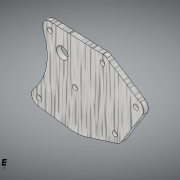
# Autodesk Inventor part: 後ろ脚内フレーム
Saved by Autodesk Inventor 2019 (Build 230136000, 136)
## iProperties
Created: 2019-09-18
Part Number: 後ろ脚内フレーム
Material: アルミニウム 7075
Document SubType Name: Modeling
Designer: tanjihayato
Density: 2.81 g/cm^3
Appearance: サテン - ブラシ仕上げ 重厚
Mass: 19.8491 g
Surface Area: 54.8854 cm^2
Volume: 7.06374 cm^3
Author: tanjihayato
Autodesk Inventor part; units mm, degrees
ref_plane "YZ Plane" through (0, 0, 0) normal (1, 0, 0) x (0, 1, 0)
ref_plane "XZ Plane" through (0, 0, 0) normal (0, 1, 0) x (-1, 0, 0)
ref_plane "XY Plane" through (0, 0, 0) normal (0, 0, 1) x (1, 0, 0)
sketch "スケッチ1" plane through (0, 0, 0) normal (0, 0, 1) x (1, 0, 0)
  circle A0 centre (-21.6908, -16.4118) radius 19.1 construction
  circle A1 centre (-58.0056, -24.4791) radius 22.1 construction
  circle A2 centre (-105.5257, -16.4118) radius 30.1 construction
  circle A3 centre (-122.6945, 30.2622) radius 1.5
  circle A4 centre (-75.5257, 23.124) radius 1.5
  circle A5 centre (-65.5257, -10.4118) radius 1.5
  circle A6 centre (-145.5257, 0.5882) radius 1.5
  circle A7 centre (-105.5257, -16.4118) radius 7.025
  circle A8 centre (-21.6908, -16.4118) radius 1.5
  arc A9 (-17.8785, -18.8026) -> (-19.2493, -12.6317) centre (-21.6908, -16.4118) ccw
  arc A10 (-61.0009, -47.384) -> (-50.9717, -46.4821) centre (-58.0056, -24.4791) ccw
  circle A11 centre (-34.2292, -36.4056) radius 1.5
  circle A12 centre (-41.5152, -3.6073) radius 1.5
  arc A13 (-39.0737, 0.1727) -> (-41.3386, 0.8892) centre (-41.5152, -3.6073) ccw
  arc A14 (-32.8589, -40.6919) -> (-30.4168, -38.7963) centre (-34.2292, -36.4056) ccw
  circle A15 centre (-79.2726, -40.4563) radius 1.5
  circle A16 centre (-79.2726, -40.4563) radius 4.5
  line L0 (-17.8785, -18.8026) -> (-30.4168, -38.7963)
  line L1 (-32.8589, -40.6919) -> (-50.9717, -46.4821)
  line L2 (-19.2493, -12.6317) -> (-39.0737, 0.1727)
  arc A17 (-149.0922, 3.3323) -> (-149.4523, -1.6098) centre (-145.5257, 0.5882) ccw
  line L3 (-149.4523, -1.6098) -> (-132.6633, -31.6026)
  line L4 (-102.3494, -47.3492) -> (-78.813, -44.9328)
  line L5 (-61.0009, -47.384) -> (-79.8561, -44.9183)
  circle A18 centre (-72.8083, -2.3784) radius 1.5
  arc A19 (-72.6317, 2.1181) -> (-76.944, -4.1523) centre (-72.8083, -2.3784) ccw
  line L6 (-41.3386, 0.8892) -> (-72.6317, 2.1181)
  arc A20 (-61.4337, -12.2841) -> (-61.2133, -9.1259) centre (-65.5257, -10.4118) ccw
  line L7 (-61.4337, -12.2841) -> (-75.1806, -42.3286)
  arc A21 (-82.5911, -37.417) -> (-76.944, -4.1523) centre (-105.5257, -16.4118) ccw
  arc A22 (-132.6633, -31.6026) -> (-102.3494, -47.3492) centre (-105.5257, -16.4118) ccw
  arc A23 (-122.0212, 34.7115) -> (-126.261, 33.0062) centre (-122.6945, 30.2622) ccw
  arc A24 (-71.2133, 24.4099) -> (-74.8523, 27.5733) centre (-75.5257, 23.124) ccw
  line L8 (-126.261, 33.0062) -> (-149.0922, 3.3323)
  line L9 (-122.0212, 34.7115) -> (-74.8523, 27.5733)
  line L10 (-71.2133, 24.4099) -> (-61.2133, -9.1259)
  circle A25 centre (-58.0056, -24.4791) radius 1.5
  point P0 (0, 0)
  point P1 (0, 0)
  dimension "d0" = 14.05
  dimension "d1" = 3
  dimension "d2" = 3
  dimension "d3" = 1
  dimension "d4" = 3
  dimension "d5" = 3
  dimension "d6" = 3
  dimension "d7" = 3
  dimension "d8" = 3
  dimension "d9" = 3
  dimension "d10" = 9
  dimension "d11" = 3
  dimension "d12" = 3
  dimension "d13" = 9
  dimension "d14" = 31.1
  dimension "d15" = 31.1
  dimension "d16" = 9
  dimension "d17" = 9
  dimension "d18" = 3
  constraints: 30 tangent, 26 centre point, 26 point on circle, 22 end point, 9 coincident
  measures "d0" diameter of A7
  measures "d1" diameter of A8
  measures "d2" radial gap between concentric circles of A8 A9
  measures "d3" radial gap between concentric circles of A1 A10
  measures "d4" diameter of A11
  measures "d5" diameter of A12
  measures "d6" radial gap between concentric circles of A12 A13
  measures "d7" radial gap between concentric circles of A11 A14
  measures "d8" diameter of A15
  measures "d9" radial gap between concentric circles of A15 A16
  measures "d10" diameter of A17
  measures "d11" diameter of A18
  measures "d12" radial gap between concentric circles of A18 A19
  measures "d13" diameter of A20
  measures "d14" radius of A22
  measures "d15" radius of A21
  measures "d16" diameter of A23
  measures "d17" diameter of A24
  measures "d18" diameter of A25
extrude "押し出し1" add sketch "スケッチ1" along normal blind 3 contours L0 A14 L1 A10 L5 L4 A16 L7 A20 L10 L6 A13 L2 A9 | L10 A20 L7 A16 A21 A19 L6 | L5 A16 L4 | A16
sketch "スケッチ2" plane through (0, 0, 0) normal (0, 0, -1) x (-1, 0, 0)
  circle A0 centre (58.0056, -24.4791) radius 1.5 projected
  circle A1 centre (72.8083, -2.3784) radius 1.5 projected
  circle A2 centre (41.5152, -3.6073) radius 1.5 projected
  circle A3 centre (34.2292, -36.4056) radius 1.5 projected
  circle A4 centre (21.6908, -16.4118) radius 1.5 projected
  circle A5 centre (65.5257, -10.4118) radius 1.5 projected
  circle A6 centre (79.2726, -40.4563) radius 1.5 projected
  arc A7 (79.8561, -44.9183) -> (82.5911, -37.417) centre (79.2726, -40.4563) ccw projected
  arc A8 (76.944, -4.1523) -> (82.5911, -37.417) centre (105.5257, -16.4118) ccw projected
  arc A9 (76.944, -4.1523) -> (72.6317, 2.1181) centre (72.8083, -2.3784) ccw projected
  line L0 (41.3386, 0.8892) -> (72.6317, 2.1181) projected
  arc A10 (41.3386, 0.8892) -> (39.0737, 0.1727) centre (41.5152, -3.6073) ccw projected
  line L1 (19.2493, -12.6317) -> (39.0737, 0.1727) projected
  arc A11 (19.2493, -12.6317) -> (17.8785, -18.8026) centre (21.6908, -16.4118) ccw projected
  line L2 (30.4168, -38.7963) -> (17.8785, -18.8026) projected
  arc A12 (30.4168, -38.7963) -> (32.8589, -40.6919) centre (34.2292, -36.4056) ccw projected
  line L3 (50.9717, -46.4821) -> (32.8589, -40.6919) projected
  arc A13 (50.9717, -46.4821) -> (61.0009, -47.384) centre (58.0056, -24.4791) ccw projected
  line L4 (79.8561, -44.9183) -> (61.0009, -47.384) projected
  circle A14 centre (65.5257, -10.4118) radius 3.5
  point P0 (0, 0)
  dimension "d21" = 7
  constraints: 1 centre point, 1 coincident
  measures "d21" diameter of A14
extrude "押し出し2" cut sketch "スケッチ2" against normal blind 10 contours A14
